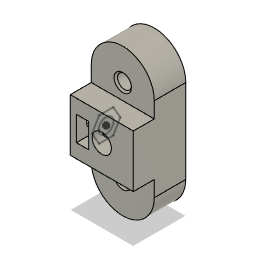
PENDRIVE inserts v1 (Autodesk Fusion 360 design; units mm, degrees)
Autodesk Fusion 360 part; units mm, degrees
note: some values were not read from the file. Set by a fixed rule: which sketch regions a step uses.
sketch "Sketch1" plane through (0, 0, 0) normal (0, 0, 1) x (1, 0, 0)
  line L0 (-9, -12) -> (-9, 12)
  line L1 (9, 12) -> (9, -12)
  line L2 (9, -21) -> (-9, 21) construction
  line L3 (-9, -21) -> (9, 21) construction
  line L4 (9, -7.5) -> (-9, -7.5)
  line L5 (-9, -7.5) -> (-9, 7.5)
  line L6 (-9, 7.5) -> (9, 7.5)
  line L7 (9, 7.5) -> (9, -7.5)
  line L8 (9, -7.5) -> (-9, 7.5) construction
  line L9 (-9, -7.5) -> (9, 7.5) construction
  circle A0 centre (0, 0) radius 2.75
  arc A1 (0, 21) -> (-9, 12) centre (0, 12) ccw
  arc A2 (9, 12) -> (0, 21) centre (0, 12) ccw
  arc A3 (0, -21) -> (9, -12) centre (0, -12) ccw
  arc A4 (-9, -12) -> (0, -21) centre (0, -12) ccw
  line L10 (0, -21.9731) -> (0, 33.0269) construction
  line L11 (2.0496, 8.45) -> (4.0992, 12)
  line L12 (4.0992, 12) -> (2.0496, 15.55)
  line L13 (2.0496, 15.55) -> (-2.0496, 15.55)
  line L14 (-2.0496, 15.55) -> (-4.0992, 12)
  line L15 (-4.0992, 12) -> (-2.0496, 8.45)
  line L16 (-2.0496, 8.45) -> (2.0496, 8.45)
  line L17 (2.0496, -15.55) -> (4.0992, -12)
  line L18 (4.0992, -12) -> (2.0496, -8.45)
  line L19 (2.0496, -8.45) -> (-2.0496, -8.45)
  line L20 (-2.0496, -8.45) -> (-4.0992, -12)
  line L21 (-4.0992, -12) -> (-2.0496, -15.55)
  line L22 (-2.0496, -15.55) -> (2.0496, -15.55)
  circle A5 centre (0, 12) radius 2
  circle A6 centre (0, -12) radius 2
  line L23 (-9, 0) -> (0, 0) construction
  line L24 (-3.75, 3.5) -> (-7.25, 3.5)
  line L25 (-7.25, 3.5) -> (-7.25, -3.5)
  line L26 (-7.25, -3.5) -> (-3.75, -3.5)
  line L27 (-3.75, -3.5) -> (-3.75, 3.5)
  line L28 (-3.75, 3.5) -> (-7.25, -3.5) construction
  line L29 (-7.25, 3.5) -> (-3.75, -3.5) construction
  point P0 (0, 12)
  point P1 (0, -12)
  point P2 (-5.5, 0)
  dimension "d14" = 18
  dimension "d15" = 42
  dimension "d16" = 18
  dimension "d17" = 15
  dimension "d18" = 5.5
  dimension "d19" = 9
  dimension "d20" = 12
  dimension "d21" = 12
  dimension "d22" = 3.55
  dimension "d23" = 3.55
  dimension "d24" = 4
  dimension "d25" = 4
  dimension "d26" = 3.5
  dimension "d27" = 7
  dimension "d28" = 3.5
  constraint parallel L0 L1
  constraint coincident L2 A0.centre
  constraint coincident L3 A0.centre
  constraint horizontal L4
  constraint perpendicular L4 L5
  constraint parallel L4 L6
  constraint parallel L5 L7
  constraint coincident L8 A0.centre
  constraint coincident L9 A0.centre
  constraint coincident A0.centre L23.end
  constraint coincident L2.end L0
  constraint tangent L0 A1
  constraint coincident L3.end L1
  constraint tangent L1 A2
  constraint equal A1 A2
  constraint coincident A1.start A2.end
  constraint coincident L2.start L1
  constraint tangent L1 A3
  constraint equal A1 A3
  constraint coincident L3.start L0
  constraint tangent L0 A4
  constraint equal A1 A4
  constraint coincident A3.start A4.end
  constraint parallel L1 L10
  constraint coincident L10 A0.centre
  constraint coincident P1 L10
  constraint coincident P0 L10
  constraint vertical L10
  constraint coincident P0 A1.centre
  constraint coincident P1 A3.centre
  constraint horizontal L19
  constraint horizontal L16
  constraint concentric A4 A6
  constraint midpoint L0 L23.start
  constraint perpendicular L10 L23
  constraint horizontal L24
  constraint perpendicular L24 L25
  constraint parallel L24 L26
  constraint parallel L25 L27
  constraint coincident L28 P2
  constraint coincident L29 P2
  constraint coincident L23 P2
  measures "d14" distance of L2.end L3.end
  measures "d15" distance of L3.start L2.end
  measures "d16" distance of L5.end L6.end
  measures "d17" distance of L4.end L5.end
  measures "d18" diameter of A0
  measures "d19" radius of A1
  measures "d20" distance of A0.centre P0
  measures "d21" distance of A0.centre P1
  measures "d22" distance of P0 L16
  measures "d23" distance of P1 L22
  measures "d24" diameter of A5
  measures "d25" diameter of A6
  measures "d26" distance of L25.end L26.end
  measures "d27" distance of L24.end L25.end
  measures "d28" distance of L5 P2
extrude "Extrude1" add sketch "Sketch1" against normal blind 5 contours L0 L1 L4 A3 A4 | L0 L1 L4 L5 L6 L7 | L0 L1 L6 A1 A2 | L11 L12 L13 L14 L15 L16 | L17 L18 L19 L20 L21 L22 | L24 L25 L26 L27
extrude "Extrude2" add sketch "Sketch1" along normal blind 10 contours L0 L1 L4 L5 L6 L7 | L24 L25 L26 L27
extrude "Extrude3" [suppressed]
extrude "Extrude7" add sketch "Sketch1" along normal blind 4 contours L0 L1 L4 A3 A4 | L0 L1 L6 A1 A2 | L11 L12 L13 L14 L15 L16 | L17 L18 L19 L20 L21 L22
extrude "Extrude4" cut sketch "Sketch1" against normal blind 5 from surface at 10 contours L24 L25 L26 L27
sketch "Sketch2" plane through (-3.75, 0, 0) normal (-1, 0, 0) x (0, 0, 1)
  line L0 (10, -3.5) -> (10, 3.5)
  line L1 (10, 3.5) -> (5, 3.5)
  line L2 (5, 3.5) -> (5, -3.5)
  line L3 (5, -3.5) -> (10, -3.5)
  line L4 (9.0415, 0) -> (7.0207, 3.5)
  line L5 (7.0207, 3.5) -> (2.9793, 3.5)
  line L6 (2.9793, 3.5) -> (0.9585, 0)
  line L7 (0.9585, 0) -> (2.9793, -3.5)
  line L8 (2.9793, -3.5) -> (7.0207, -3.5)
  line L9 (7.0207, -3.5) -> (9.0415, 0)
  circle A0 centre (5, 0) radius 2.1
  point P0 (5, 0)
  dimension "d38" = 3.5
  dimension "d41" = 4.2
  constraint midpoint L2 P0
  constraint horizontal L5
  constraint coincident P0 A0.centre
  measures "d38" distance of P0 L9
  measures "d41" diameter of A0
extrude "Extrude5" cut sketch "Sketch2" along normal up to surface (3.5 mm away) contours L1 L2 L3 L4 L5 L8 L9 A0 | L2 L5 L6 L7 L8 A0 | L2 A0 | L2 A0
extrude "Extrude6" cut sketch "Sketch2" against normal blind 9 from surface at 5.25 contours L2 A0 | L2 A0
chamfer "Chamfer1" [suppressed]
chamfer "Chamfer2" distance 0.5 angle 45 2 edges at (-1.8647, 12.7232, 4) (-1.8647, -11.2768, 4)
